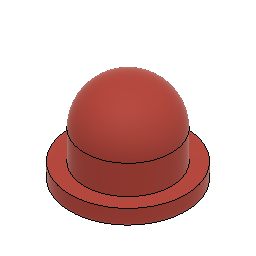
Translucent Light Pipe v2 (Autodesk Fusion 360 design; units mm, degrees)
Autodesk Fusion 360 part; units mm, degrees
sketch "Sketch1" plane through (0, 0, 0) normal (0, 1, 0) x (1, 0, 0)
  circle A0 centre (0, 0) radius 1.5
  circle A1 centre (0, 0) radius 2
  dimension "d1" = 3
  dimension "d2" = 4
  constraint coincident A0.centre A1.centre
  constraint concentric A0 A1
  measures "d1" diameter of A0
  measures "d2" diameter of A1
extrude "Extrude1" add sketch "Sketch1" along normal blind 0.5 contours A0 | A1
extrude "Extrude2" add sketch "Sketch1" along normal blind 1.5 contours A0
sphere "SpherePrimitive1" add diameter 3 placed x (-1, 0, 0) y (0, 0, 1) z (0, 1, 0) at (0, 1.5, 0)
